Barrel Rotary Mount Center Spacer_v3 (Autodesk Fusion 360 design; units mm, degrees)
Autodesk Fusion 360 part; units mm, degrees
sketch "Sketch1" plane through (0, 0, 0) normal (1, 0, 0) x (0, 1, 0)
  line L0 (0, 0) -> (5.6, 0)
  line L1 (2.8, 0) -> (2.8, 6) construction
  line L2 (2.8, 6) -> (-0.2, 6)
  line L3 (2.8, 6) -> (5.8, 6)
  line L4 (-0.2, 6) -> (-0.2, 3)
  line L5 (-0.2, 3) -> (0, 0)
  line L6 (5.8, 6) -> (5.8, 3)
  line L7 (5.8, 3) -> (5.6, 0)
  dimension "d1" = 5.6
  dimension "d2" = 3
  dimension "d3" = 3
  constraint coincident L0.start L5.end
  constraint horizontal L0
  constraint midpoint L0 L1.start
  constraint perpendicular L0 L1
  constraint perpendicular L1 L2
  constraint perpendicular L1 L3
  constraint perpendicular L2 L4
  constraint perpendicular L3 L6
  measures "d1" distance of L0.start L0.end
  measures "d2" distance of L1.end L2.end
  measures "d3" distance of L1.end L3.end
extrude "Extrude1" add sketch "Sketch1" along normal blind 52.4
